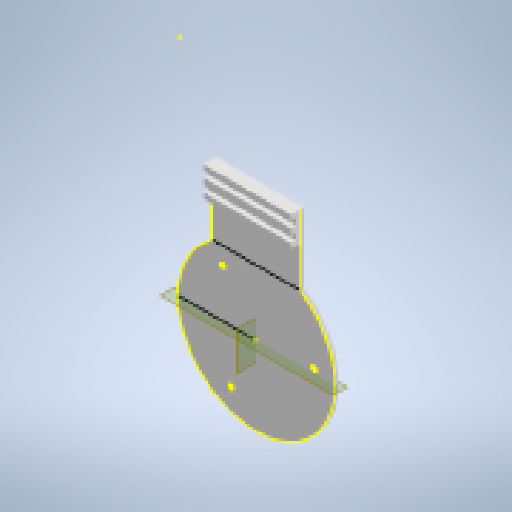
# Autodesk Inventor part: AnemoHolder
Saved by Autodesk Inventor 2023 (Build 270158000, 158)
## iProperties
Created: 2023-03-27
Part Number: AnemoHolder
Material: Générique
Document SubType Name: Modeling
Designer: eleves
Density: 1 g/cm^3
Appearance: Par défaut
Author: eleves
## iProperties of the stored document rainHolder_Impression 3D.ipt
Created: 2023-03-27
Part Number: rainHolder_Impression 3D
Material: Générique
Document SubType Name: Modeling
Designer: eleves
Density: 1 g/cm^3
Appearance: Par défaut
Author: eleves
Autodesk Inventor part; units mm, degrees
ref_plane "YZ Plane" through (0, 0, 0) normal (1, 0, 0) x (0, 1, 0)
ref_plane "XZ Plane" through (0, 0, 0) normal (0, 1, 0) x (-1, 0, 0)
ref_plane "XY Plane" through (0, 0, 0) normal (0, 0, 1) x (1, 0, 0)
sketch "Esquisse1" plane through (0, 0, 0) normal (0, 0, 1) x (1, 0, 0)
  line L0 (-65.5174, -57.3571) -> (-65.5174, -54.3571) construction
  line L1 (-65.5174, -57.3571) -> (68.5174, -57.3571) construction
  line L2 (68.5174, -54.3571) -> (68.5174, -57.3571) construction
  line L3 (68.5174, -54.3571) -> (-65.5174, -54.3571) construction
  line L4 (-65.5174, -65.3571) -> (-65.5174, -62.3571) construction
  line L5 (-65.5174, -65.3571) -> (68.5174, -65.3571) construction
  line L6 (68.5174, -62.3571) -> (68.5174, -65.3571) construction
  line L7 (68.5174, -62.3571) -> (-65.5174, -62.3571) construction
  line L8 (68.5174, -54.3571) -> (-65.5174, -65.3571) construction
  line L9 (-65.5174, -54.3571) -> (68.5174, -65.3571) construction
  line L10 (-65.5174, -61.8571) -> (68.5174, -61.8571)
  line L11 (68.5174, -61.8571) -> (68.5174, -57.8571)
  line L12 (68.5174, -57.8571) -> (-65.5174, -57.8571)
  line L13 (-65.5174, -57.8571) -> (-65.5174, -61.8571)
  line L14 (-65.5174, -61.8571) -> (68.5174, -57.8571) construction
  line L15 (68.5174, -61.8571) -> (-65.5174, -57.8571) construction
  line L16 (68.5174, -54.3571) -> (18.5174, -54.3571)
  line L17 (18.5174, -54.3571) -> (18.5174, -51.3571)
  line L18 (18.5174, -51.3571) -> (68.5174, -51.3571)
  line L19 (68.5174, -51.3571) -> (68.5174, -54.3571)
  line L20 (68.5174, -65.3571) -> (18.5174, -65.3571)
  line L21 (18.5174, -65.3571) -> (18.5174, -68.3571)
  line L22 (18.5174, -68.3571) -> (68.5174, -68.3571)
  line L23 (68.5174, -68.3571) -> (68.5174, -65.3571)
  line L24 (18.5174, -57.8571) -> (18.5174, -61.8571)
  point P0 (0, 0)
  point P1 (1.5, -59.8571)
  dimension "d1" = 0.5
  dimension "d2" = 50
  dimension "d3" = 3
  dimension "d4" = 3
  constraints: 34 end point, 6 parallel, 4 perpendicular, 3 horizontal, 3 midpoint, 3 point on line
  measures "d1" distance between parallel lines of L1 L12
  measures "d2" distance of L17.end L18.end
  measures "d3" distance of L18.end L2.start
  measures "d4" distance of L22.end L5.end
extrude "Extrusion1" add sketch "Esquisse1" along normal blind 2.9 contours L24 L12 L11 L10 | L16 L17 L18 L19 | L23 L22 L21 L20
sketch "Esquisse13" plane through (0, 0, 0) normal (0, 0, -1) x (-1, 0, 0)
  line L0 (-68.5174, -68.3571) -> (-68.5174, -65.3571) projected
  line L1 (-18.5174, -51.3571) -> (-68.5174, -51.3571)
  line L2 (-68.5174, -51.3571) -> (-68.5174, -68.3571)
  line L3 (-68.5174, -68.3571) -> (-18.5174, -68.3571)
  line L4 (-18.5174, -68.3571) -> (-18.5174, -51.3571)
  point P0 (0, 0)
  constraints: 8 end point, 2 parallel, 1 horizontal, 1 perpendicular
extrude "Extrusion12" add sketch "Esquisse13" along normal blind 2
sketch "Esquisse24" plane through (0, 0, -2) normal (0, 0, -1) x (-1, 0, 0)
  line L0 (-18.5174, -65.3571) -> (-18.5174, -68.3571) projected
  line L1 (-18.5174, -51.3571) -> (-68.5174, -51.3571) projected
  line L2 (-18.5174, -68.3571) -> (-68.5174, -68.3571)
  line L3 (-68.5174, -68.3571) -> (-68.5174, -51.3571)
  line L4 (-68.5174, -51.3571) -> (-18.5174, -51.3571)
  line L5 (-18.5174, -51.3571) -> (-18.5174, -68.3571)
  point P0 (0, 0)
  constraints: 8 end point, 2 parallel, 1 horizontal, 1 perpendicular
extrude "Extrusion21" add sketch "Esquisse24" along normal blind 5
sketch "Esquisse25" plane through (18.5174, -68.3571, 2.9) normal (0, -1, 0) x (1, 0, 0)
  line L0 (50, -9.9) -> (50, 0) projected
  line L1 (50, -9.9) -> (0, -9.9)
  line L2 (0, -9.9) -> (0, -4.95)
  line L3 (0, -4.95) -> (50, -4.95)
  line L4 (50, -4.95) -> (50, -9.9)
  line L5 (0, -9.9) -> (0, 0) construction
  point P0 (-18.5174, -2.9)
  constraints: 8 end point, 2 parallel, 1 collinear, 1 horizontal, 1 perpendicular
extrude "Extrusion22" add sketch "Esquisse25" along normal blind 15
sketch "Esquisse26" plane through (18.5174, -68.3571, -2.05) normal (0, 0, 1) x (1, 0, 0)
  line L0 (50, -15) -> (0, -15) projected
  line L1 (0, 0) -> (50, 0) projected
  line L2 (0, -15) -> (50, 0)
  line L3 (0, 0) -> (50, -15)
  line L4 (25, -7.5) -> (25, -60)
  circle A0 centre (25, -60) radius 45
  line L5 (0, -15) -> (50, -15) projected
  line L6 (0, -15) -> (0, -22.5834)
  line L7 (50, 0) -> (50, -15) projected
  line L8 (50, -15) -> (50, -22.5834)
  line L9 (0, -15) -> (25, -15)
  line L10 (25, -15) -> (50, -15)
  point P0 (-18.5174, 68.3571)
  dimension "d89" = 90
  constraints: 14 end point, 3 point on circle, 2 collinear, 2 midpoint, 2 tangent, 1 centre point, 1 coincident, 1 perpendicular, 1 vertical
  measures "d89" diameter of A0
extrude "Extrusion23" add sketch "Esquisse26" against normal up to surface (4.95 mm away) contours L8 A0 L0 | A0 L6 L0 | A0
sketch "Esquisse27" plane through (0, 0, -7) normal (0, 0, -1) x (-1, 0, 0)
  line L0 (-18.5174, -51.3571) -> (-18.5174, -90.9406) projected
  line L1 (-18.5174, -51.3571) -> (-68.5174, -51.3571) projected
  line L2 (-68.5174, -51.3571) -> (-68.5174, -90.9406) projected
  arc A0 (-68.5174, -90.9406) -> (-18.5174, -90.9406) centre (-43.5174, -128.3571) ccw projected
  point P0 (0, 0)
extrude "Extrusion24" cut sketch "Esquisse27" against normal blind 2.5
sketch "Esquisse28" plane through (18.5174, -68.3571, -2.05) normal (0, 0, 1) x (1, 0, 0)
  arc A0 (0, -22.5834) -> (50, -22.5834) centre (25, -60) ccw construction
  line L0 (25, -60) -> (-20, -60)
  point P0 (-18.5174, 68.3571)
  constraints: 2 end point, 1 horizontal, 1 point on circle
ref_plane "Plan de construction5" through (43.5174, -128.3571, -2.05) normal (0, -1, 0) x (1, 0, 0)
ref_plane "Plan de construction6" through (43.5174, -128.3571, -2.05) normal (-1, 0, 0) x (0, -1, 0)
sketch "Esquisse29" plane through (0, 0, -4.5) normal (0, 0, -1) x (-1, 0, 0)
  circle A0 centre (-29.1178, -158.4374) radius 1.5 projected
  circle A1 centre (-24.1083, -100.8982) radius 1.5 projected
  circle A2 centre (-76.4793, -125.6998) radius 1.5 projected
  point P0 (0, 0)
extrude "Extrusion25" cut sketch "Esquisse29" against normal blind 15
sketch "Esquisse30" plane through (18.5174, -68.3571, -2.05) normal (0, 0, 1) x (1, 0, 0)
  circle A0 centre (57.9619, -57.3427) radius 1.5 projected
  circle A1 centre (10.6003, -90.0802) radius 1.5 projected
  circle A2 centre (5.5909, -32.541) radius 1.5 projected
  line L0 (0, 0) -> (50, 0) projected
  line L1 (0, 0) -> (0, -22.5834) projected
  arc A3 (0, -22.5834) -> (50, -22.5834) centre (25, -60) ccw projected
  line L2 (50, 0) -> (50, -22.5834) projected
  line L3 (50, -22.5834) -> (50, 17) projected
  line L4 (50, -22.5834) -> (0, -22.5834)
  point P0 (-18.5174, 68.3571)
  point P1 (0, -22.5834)
  constraints: 2 end point, 1 horizontal
extrude "Extrusion26" add sketch "Esquisse30" along normal blind 10 contours L4 A3
sketch "Esquisse31" plane through (0, 0, -4.5) normal (0, 0, -1) x (-1, 0, 0)
  line L0 (-97.6483, -128.3571) -> (22.3325, -128.3571) projected
  line L1 (-43.5174, -178.8817) -> (-43.5174, -79.6766) projected
  circle A0 centre (-43.5174, -128.3571) radius 43
  arc A1 (-68.5174, -90.9406) -> (-18.5174, -90.9406) centre (-43.5174, -128.3571) ccw projected
  line L2 (-68.5174, -68.3571) -> (-68.5174, -90.9406) projected
  line L3 (-68.5174, -90.9406) -> (-18.5174, -90.9406)
  point P0 (0, 0)
  point P1 (-64.707, -90.9406)
  point P2 (-22.3278, -90.9406)
  dimension "d98" = 2
  constraints: 2 end point, 2 point on line, 1 centre point, 1 perpendicular
  measures "d98" radial gap between concentric circles of A1 A0
sketch "Esquisse34" plane through (18.5174, -68.3571, 7.95) normal (0, 0, 1) x (1, 0, 0)
  arc A0 (0, -22.5834) -> (50, -22.5834) centre (25, -60) ccw projected
  line L0 (50, -22.5834) -> (0, -22.5834) projected
  circle A1 centre (5.5909, -32.541) radius 1.5 projected
  circle A2 centre (10.6003, -90.0802) radius 1.5 projected
  circle A3 centre (57.9619, -57.3427) radius 1.5 projected
  arc A4 (0.6142, -24.5834) -> (49.3858, -24.5834) centre (25, -60) ccw
  line L1 (0.6142, -24.5834) -> (49.3858, -24.5834)
  point P0 (-18.5174, 68.3571)
  dimension "d103" = 2
  constraints: 2 end point, 2 point on circle, 1 centre point, 1 other
  measures "d103" radial gap between concentric circles of A0 A4
extrude "Extrusion29" cut sketch "Esquisse34" against normal blind 10 contours L1 A4
sketch "Esquisse35" plane through (43.5174, -128.3571, -2.05) normal (-1, 0, 0) x (0, -1, 0)
  line L0 (0, 9.1389) -> (0, 21.1265) construction
  circle A0 centre (0, 15.1327) radius 2
  point P0 (-128.3571, 2.05)
  dimension "d106" = 4
  constraints: 2 end point, 1 centre point, 1 midpoint, 1 vertical
  measures "d106" diameter of A0
